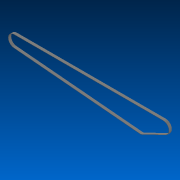
# Autodesk Inventor part: 225T x 9mm Wide Timing Belt (HTD 5mm)(217-3469)
Saved by Autodesk Inventor 2022 (Build 260153000, 153)
## iProperties
Created: 2022-01-07
Part Number: 225T x 9mm Wide Timing Belt (HTD 5mm)(217-3469)
Material: Fiberglass Batt
Document SubType Name: Modeling
Designer: omard
Density: 0.032 g/cm^3
Appearance: Gray
Author: omard
Autodesk Inventor part; units mm, degrees
ref_plane "YZ Plane" through (0, 0, 0) normal (1, 0, 0) x (0, 1, 0)
ref_plane "XZ Plane" through (0, 0, 0) normal (0, 1, 0) x (-1, 0, 0)
ref_plane "XY Plane" through (0, 0, 0) normal (0, 0, 1) x (1, 0, 0)
sketch "Sketch1" plane through (0, 0, 0) normal (0, 0, 1) x (1, 0, 0)
  arc A0 (0, 19.1008) -> (-1.7113, -19.024) centre (0, 0) ccw
  arc A1 (495.3, -19.1008) -> (503.6151, -17.1959) centre (495.3, 0) ccw construction
  line L0 (0, 19.1008) -> (495.3, 19.1008)
  line L1 (495.3, -19.1008) -> (0, -19.1008) construction
  line L2 (495.3, 20.1008) -> (0, 20.1008)
  arc A2 (0, 20.1008) -> (-1.8009, -20.02) centre (0, 0) ccw
  line L3 (0, -20.1008) -> (495.3, -20.1008) construction
  arc A3 (495.3, -20.1008) -> (497.9784, -19.9215) centre (495.3, 0) ccw construction
  arc A4 (418.1044, -56.7878) -> (423.9376, -55.7243) centre (419.1, -45.72) ccw
  arc A5 (418.0148, -57.7838) -> (424.3729, -56.6245) centre (419.1, -45.72) ccw
  line L4 (424.3729, -56.6245) -> (504.0505, -18.0962)
  line L5 (503.6151, -17.1959) -> (423.9376, -55.7243)
  line L6 (418.0148, -57.7838) -> (-1.8009, -20.02)
  line L7 (-1.7113, -19.024) -> (418.1044, -56.7878)
  arc A6 (497.9784, -19.9215) -> (504.0505, -18.0962) centre (495.3, 0) ccw construction
  arc A7 (504.0505, -18.0962) -> (495.3, 20.1008) centre (495.3, 0) ccw
  arc A8 (503.6151, -17.1959) -> (495.3, 19.1008) centre (495.3, 0) ccw
  arc A9 (-1.7113, -19.024) -> (0, -19.1008) centre (0, 0) ccw construction
  arc A10 (-1.8009, -20.02) -> (0, -20.1008) centre (0, 0) ccw construction
  dimension "d0" = 495.3
  dimension "d1" = 38.2016
  dimension "d2" = 1
  dimension "d5" = 22.225
  dimension "d6" = 76.2
  dimension "d7" = 45.72
  constraints: 25 tangent, 23 point on circle, 16 end point, 11 centre point, 2 coincident, 1 equal radius, 1 horizontal alignment, 1 parallel, 1 point on line
  measures "d0" distance of A1.centre point (0, 0)
  measures "d1" diameter of A1
  measures "d2" distance between parallel lines of L0 L2
  measures "d5" diameter of A4
  measures "d6" horizontal distance of A4.centre A1.centre
  measures "d7" vertical distance of A1.centre A4.centre
extrude "Extrusion1" add sketch "Sketch1" along normal mid plane 9
body "Solid1"
